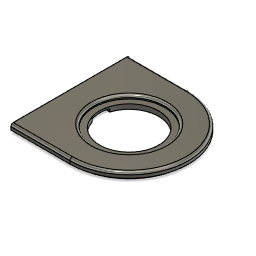
pot cover v5 (Autodesk Fusion 360 design; units mm, degrees)
Autodesk Fusion 360 part; units mm, degrees
sketch "スケッチ1" plane through (0, 0, 0) normal (0, 1, 0) x (1, 0, 0)
  line L0 (84.9076, 0) -> (-96.0768, 0) construction
  line L1 (0, -64.1732) -> (0, 68.3912) construction
  line L2 (0, -50) -> (-50, -50)
  line L3 (-50, -50) -> (-50, 50)
  line L4 (0, 50) -> (-50, 50)
  circle A0 centre (0, 0) radius 25
  arc A1 (0, -50) -> (0, 50) centre (0, 0) ccw
  line L5 (0, -47) -> (-50, -47)
  line L6 (0, 47) -> (-50, 47)
  arc A2 (0, -47) -> (0, 47) centre (0, 0) ccw
  circle A3 centre (0, 0) radius 30
  line L7 (-50, -47) -> (-52, -47)
  line L8 (-52, -47) -> (-52, 47)
  line L9 (-52, 47) -> (-50, 47)
  line L10 (-50, 47) -> (-50, -47)
  line L11 (-31.5, 57.8245) -> (-31.5, -58.1462) construction
  line L12 (-37.5, -7.5) -> (-25, -7.5)
  line L13 (-25, 7.5) -> (-37.5, 7.5)
  line L14 (-37.5, 7.5) -> (-37.5, -7.5)
  line L15 (-25, -7.5) -> (-23.8485, -7.5)
  line L16 (-25, 7.5) -> (-23.8485, 7.5)
  line L17 (-32.1391, -10) -> (-28.2843, -10) construction
  line L18 (-32.1391, 10) -> (-28.2843, 10) construction
  circle A4 centre (-31.5, -10) radius 1.35
  circle A5 centre (-31.5, 10) radius 1.35
  line L19 (-52, -27) -> (-50, -27.0394)
  line L20 (-52, 27) -> (-50, 27)
  dimension "d1" = 100
  dimension "d2" = 50
  dimension "d3" = 50
  dimension "d4" = 94
  dimension "d5" = 60
  dimension "d17" = 2
  dimension "d18" = 31.5
  dimension "d20" = 15
  dimension "d21" = 7.5
  dimension "d22" = 6
  dimension "d23" = 20
  dimension "d24" = 10
  dimension "d25" = 2.7
  dimension "d26" = 2.7
  dimension "d36" = 20
  dimension "d37" = 20
  constraint horizontal L0
  constraint perpendicular L0 L1
  constraint coincident A0.centre A1.centre
  constraint coincident L1 L2.start
  constraint tangent L2 A1
  constraint perpendicular L0 L3
  constraint coincident L1 L4.start
  constraint coincident L3 L4.end
  constraint tangent L4 A1
  constraint concentric A0 A1
  constraint concentric A1 A2
  constraint coincident L1 L5.start
  constraint coincident L3 L5.end
  constraint tangent L5 A2
  constraint coincident L1 L6.start
  constraint coincident L3 L6.end
  constraint tangent L6 A2
  constraint concentric A2 A3
  constraint horizontal L7
  constraint vertical L8
  constraint horizontal L9
  constraint vertical L10
  constraint perpendicular L2 L11
  constraint horizontal L12
  constraint horizontal L13
  constraint vertical L14
  constraint coincident A0 L15.end
  constraint coincident A0 L16.end
  constraint collinear L12 L15
  constraint collinear L13 L16
  constraint coincident A3 L17.end
  constraint perpendicular L11 L17
  constraint coincident A3 L18.end
  constraint perpendicular L11 L18
  constraint coincident L17 A4.centre
  constraint coincident L11 A4.centre
  constraint coincident L11 A5.centre
  constraint coincident L18 A5.centre
  constraint coincident L8 L19.start
  constraint coincident L3 L19.end
  constraint coincident L8 L20.start
  constraint coincident L10 L20.end
  constraint perpendicular L10 L20
  constraint collinear L6 L9
  measures "d1" diameter of A1
  measures "d2" distance of L2.start L2.end
  measures "d3" diameter of A0
  measures "d4" diameter of A2
  measures "d5" diameter of A3
  measures "d17" distance of L3 L8
  measures "d18" distance of L1 L11
  measures "d20" distance of L12 L13
  measures "d21" distance of L0 L12
  measures "d22" distance of L11 L14
  measures "d23" distance of L17 L18
  measures "d24" distance of L0 L18
  measures "d25" diameter of A4
  measures "d26" diameter of A5
  measures "d36" vertical distance of L5.end L19.start
  measures "d37" distance of L6.end L20.end
extrude "押し出し1" add sketch "スケッチ1" along normal blind 5 contours L2 L3 L4 A1 L5 L6 A2 | L3 L5 L6 A2 L10 | A3 L12 L13 L14 | A4 | A5
fillet "フィレット1" radius 2 3 edges at (-25, 5, 50) (50, 5, 0) (-25, 5, -50)
fillet "フィレット2" radius 2 1 edges at (-27.9698, 5, -10.8485)
extrude "押し出し3" add sketch "スケッチ1" against normal blind 2 contours L3 L7 L8 L10 L19 | L3 L5 L6 A2 L10 | L3 L8 L10 L19 L20 | L3 L8 L9 L10 L20 | A0 A3 L12 L13 L15 L16 | A0 A3 L12 L13 L15 L16 | A3 L12 L13 L14 | A4 | A5
extrude "押し出し7" add sketch "スケッチ1" along normal blind 2 contours A0 A3 L12 L13 L15 L16 | A0 A3 L12 L13 L15 L16
extrude "押し出し8" cut 1 faces at (-33.3333, 0, -49) along direction (0, 1, 0) blind 0.5
extrude "押し出し9" cut 1 faces at (-50.6667, 0, 15.6667) along direction (0, -1, 0) blind 0.5
extrude "押し出し4" cut sketch "スケッチ1" along normal blind 2.5 from surface at -2 contours A0 A3 L12 L13 L15 L16 | A3 L12 L13 L14 picked at (-28.2382, -1.7675)
extrude "押し出し5" add sketch "スケッチ1" along normal blind 3 from surface at -2 contours A4 | A5
extrude "押し出し6" cut sketch "スケッチ1" along normal blind 5 from surface at -2 contours L3 L7 L8 L10 L19 | L3 L8 L9 L10 L20 | A4 | A5
equation "d21 = d20 / 2"
equation "d24 = d23 / 2"
